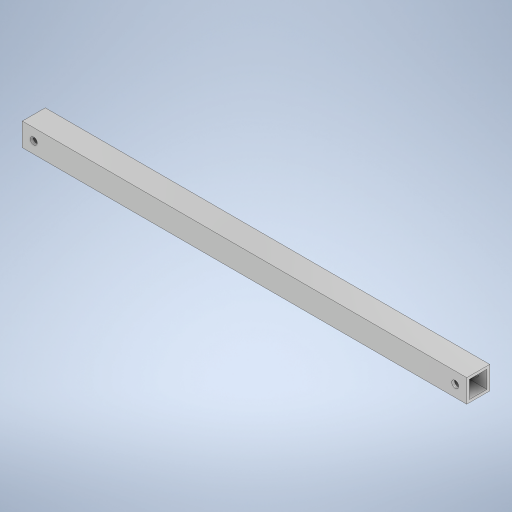
# Autodesk Inventor part: truss_1010_zegi
Saved by Autodesk Inventor 2023 (Build 270158000, 158)
## iProperties
Created: 2022-12-20
Part Number: truss_1010_zegi
Material: アルミニウム 6061-AHC
Document SubType Name: Modeling
Designer: zegi
Density: 2.7 g/cm^3
Appearance: アルミニウム - ダーク
Author: zegi
Autodesk Inventor part; units mm, degrees
ref_plane "YZ Plane" through (0, 0, 0) normal (1, 0, 0) x (0, 1, 0)
ref_plane "XZ Plane" through (0, 0, 0) normal (0, 1, 0) x (-1, 0, 0)
ref_plane "XY Plane" through (0, 0, 0) normal (0, 0, 1) x (1, 0, 0)
sketch "スケッチ2" plane through (0, 0, 0) normal (0, 0, 1) x (1, 0, 0)
  line L0 (0, 0) -> (148.4693, 71.9851)
  line L1 (148.4693, 71.9851) -> (183.3712, 0)
  line L2 (0, 0) -> (183.3712, 0)
  line L3 (-5, -5) -> (188.3712, -5)
  line L4 (188.3712, -5) -> (188.3712, 5)
  line L5 (188.3712, 5) -> (-5, 5)
  line L6 (-5, 5) -> (-5, -5)
  dimension "d3" = 165
  dimension "d4" = 80
  dimension "d5" = 10
  dimension "d6" = 5
  dimension "d7" = 5
  constraints: 14 end point, 2 coincident, 2 horizontal, 2 parallel, 2 perpendicular, 1 other
  measures "d3" distance of L0.start L0.end
  measures "d4" distance of L0.end L1.end
  measures "d5" distance of L5.end L3.start
  measures "d6" distance from line of L6 L0.start
  measures "d7" distance from line of L1.end L4
extrude "押し出し1" add sketch "スケッチ2" along normal blind 10 contours L2 L1 L5 L4 L3 L6 L0 | L0 L5 L1 L2
sketch "スケッチ3" plane through (188.3712, -5, 0) normal (1, 0, 0) x (0, 0, -1)
  line L0 (0, 0) -> (0, 10) projected
  line L1 (0, 10) -> (-10, 10) projected
  line L2 (-10, 0) -> (-10, 10) projected
  line L3 (0, 0) -> (-10, 0) projected
  line L4 (-8.8, 8.8) -> (-1.2, 8.8)
  line L5 (-1.2, 8.8) -> (-1.2, 1.2)
  line L6 (-1.2, 1.2) -> (-8.8, 1.2)
  line L7 (-8.8, 1.2) -> (-8.8, 8.8)
  point P0 (0, 5)
  dimension "d10" = 1.2
  constraints: 8 end point, 3 other
  measures "d10" distance between parallel lines of L1 L4
extrude "押し出し2" cut sketch "スケッチ3" against normal through all contours L4 L5 L6 L7
hole "穴1" at (0, 0, 0) at (183.3712, 0, 0) direction (0, 0, 1) diameter 3 end through all
